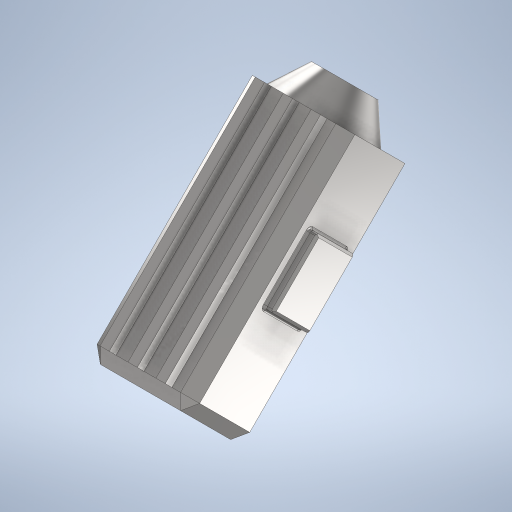
# Autodesk Inventor part: screwdriver
Saved by Autodesk Inventor 2023 (Build 270158000, 158)
## iProperties
Created: 2023-11-21
Part Number: screwdriver
Material: Steel, Mild
Document SubType Name: Modeling
Designer: Beatrice
Density: 7.85 g/cm^3
Appearance: Semi-Polished
Author: Beatrice
Autodesk Inventor part; units mm, degrees
ref_plane "YZ Plane" through (0, 0, 0) normal (1, 0, 0) x (0, 1, 0)
ref_plane "XZ Plane" through (0, 0, 0) normal (0, 1, 0) x (-1, 0, 0)
sketch "Sketch1" plane through (0, 0, 0) normal (1, 0, 0) x (0, 1, 0)
  line L0 (-19.1091, 33.3894) -> (19.1091, 33.3894) construction
  line L1 (-2.4562, 42.2517) -> (-3.9425, 12.3724) construction
  line L2 (-15.9499, 49.3393) -> (15.9499, 17.4395) construction
  line L3 (-15.9953, 17.3941) -> (15.9953, 49.3847) construction
  line L4 (-4.2099, 47.2514) -> (-6.25, 6.2414) construction
  line L5 (17.609, 51.9698) -> (-38.9081, 36.826) construction
  line L6 (18.2302, 47.2514) -> (-40.2807, 47.2514) construction
  line L7 (-2.4567, 42.2414) -> (2.4677, 42.2414) construction
  circle A0 centre (0, 47.2514) radius 3 construction
  ellipse E0 centre (0, 47.2514) end of major axis (4.2185, 47.2514) minor radius 4.2127 (4.2185, 47.2514) -> (-4.2185, 47.2514) ccw construction
  circle A1 centre (0, 47.2514) radius 4.2185 construction
  line L8 (2.4672, 42.2517) -> (-2.4562, 42.2517) construction
  line L9 (4.2215, 47.2514) -> (6.2448, 6.4952) construction
  line L10 (2.4672, 42.2517) -> (3.9506, 12.3724) construction
  line L11 (0.0006, 41.0008) -> (0, 41.0008) construction
  line L12 (-1.0918, 51.3262) -> (1.0918, 43.1767) construction
  line L13 (1.0918, 43.1767) -> (-27.4928, 38.1364) construction
  line L14 (0, 43.0329) -> (-28.9151, 45.5627) construction
  line L15 (-1.0918, 51.3262) -> (-28.367, 41.3989) construction
  line L16 (0, 51.4699) -> (-28.9151, 48.9402) construction
  line L17 (0.0006, 41.0001) -> (0, 41.0001) construction
  ellipse E1 centre (0, 47.2514) end of major axis (-3, 47.2514) minor radius 3 (0.0225, 44.2515) -> (-0.0225, 44.2515) ccw construction
  line L18 (-4.2185, 47.2514) -> (-4.2099, 47.2514) construction
  line L19 (-3.9425, 12.3724) -> (3.9506, 12.3724) construction
  ellipse E2 centre (0, 6.2414) end of major axis (6.25, 6.2414) minor radius 6.2414 (-6.2423, 6.5518) -> (6.2393, 6.6057) ccw construction
  ellipse E3 centre (0, 6.2414) end of major axis (-5, 6.2414) minor radius 5 construction
  line L20 (-6.0016, 11.2344) -> (6.0096, 11.2344) construction
  line L21 (3, 47.2514) -> (4.2185, 47.2514) construction
  line L22 (0, 48.3894) -> (0, 48.3894) construction
  line L23 (0, 51.4699) -> (0, 43.0329) construction
  line L24 (-28.9151, 45.5627) -> (-28.9151, 48.9402) construction
  line L25 (-9.1941, 44.3513) -> (-8.3969, 45.6327) construction
  circle A2 centre (-9.1612, 46.1081) radius 0.5 construction
  circle A3 centre (-9.1612, 46.1081) radius 0.9 construction
  line L26 (-9.1941, 44.3513) -> (-10.078, 43.4674) construction
  line L27 (-10.9619, 46.119) -> (-9.6062, 46.8904) construction
  line L28 (-10.9619, 46.119) -> (-9.1941, 44.3513) construction
  line L29 (-10.9619, 42.5835) -> (-10.078, 43.4674) construction
  line L30 (-11.8457, 45.2351) -> (-10.9619, 46.119) construction
  line L31 (-11.8457, 45.2351) -> (-12.7296, 44.3513) construction
  line L32 (-12.7296, 44.3513) -> (-10.9619, 42.5835) construction
  line L33 (-10.9619, 42.5835) -> (-12.2433, 41.7864) construction
  line L34 (-12.7296, 44.3513) -> (-13.501, 42.9956) construction
  line L35 (-13.4028, 41.8664) -> (-9.1612, 46.1081) construction
  circle A4 centre (-12.7187, 42.5506) radius 0.5 construction
  circle A5 centre (-12.7187, 42.5506) radius 0.9 construction
  line L36 (-27.4928, 38.1364) -> (-28.367, 41.3989) construction
  line L37 (-21.5614, 39.1823) -> (-22.7073, 43.4588) construction
  line L38 (-27.6711, 38.8017) -> (-21.8755, 40.3546) construction
  line L39 (-28.1887, 40.7336) -> (-22.3931, 42.2865) construction
  line L40 (-34.0028, 47.2514) -> (-25.2783, 38.5269) construction
  line L41 (-28.1887, 40.7336) -> (-33.0183, 39.4395) construction
  line L42 (-33.0183, 39.4395) -> (-32.5007, 37.5076) construction
  line L43 (-32.5007, 37.5076) -> (-27.6711, 38.8017) construction
  circle A6 centre (-32.7595, 38.4736) radius 1.01 construction
  circle A7 centre (-32.7595, 38.4736) radius 0.6398 construction
  line L44 (-42.8892, 48.6033) -> (-22.6298, 28.3438) construction
  circle A8 centre (-32.7595, 38.4736) radius 0.6398
  circle A9 centre (-32.7595, 38.4736) radius 1.25
  line L45 (-33.6434, 39.3574) -> (-31.8756, 37.5897)
  line L46 (-31.8756, 37.5897) -> (-33.2898, 36.1755)
  line L47 (-33.2898, 36.1755) -> (-35.0576, 37.9432)
  line L48 (-35.0576, 37.9432) -> (-33.6434, 39.3574)
  circle A10 centre (-33.0183, 39.4395) radius 0.2
  circle A11 centre (-33.7254, 38.2147) radius 0.2
  circle A12 centre (-32.5007, 37.5076) radius 0.2
  circle A13 centre (-31.7936, 38.7324) radius 0.2
  line L49 (-31, 33.8856) -> (-41.6066, 44.4922)
  line L50 (-44.7369, 41.362) -> (-34.1303, 30.7554)
  line L51 (-34.1303, 30.7554) -> (-31, 33.8856)
  line L52 (-33.6434, 39.3574) -> (-35.4365, 38.3222)
  line L53 (-33.6434, 39.3574) -> (-31.5728, 39.3574) construction
  line L54 (-31.8756, 37.5897) -> (-32.9109, 35.7965)
  line L55 (-35.4365, 38.3222) -> (-32.9109, 35.7965)
  line L56 (-32.9109, 35.7965) -> (-33.8666, 34.8408)
  line L57 (-33.8666, 34.8408) -> (-36.3923, 37.3664)
  line L58 (-36.3923, 37.3664) -> (-35.4365, 38.3222)
  line L59 (-41.6066, 44.4922) -> (-44.7369, 41.362)
  line L60 (-43.1717, 42.9271) -> (-32.5651, 32.3205) construction
  line L61 (-43.1717, 42.9271) -> (-45.2366, 44.992) construction
  line L62 (-33.5967, 46.8453) -> (-44.9671, 35.4748) construction
  circle A14 centre (-40.3433, 40.0987) radius 0.85
  line L63 (-50.4924, 41.0001) -> (-32.6081, 23.1158) construction
  line L64 (-50.4924, 41.0001) -> (-25.2002, 41.0001) construction
  line L65 (-46.7349, 37.2426) -> (-43.1994, 33.7071)
  line L66 (-43.1994, 33.7071) -> (-34.4479, 42.4585)
  line L67 (-34.4479, 42.4585) -> (-37.9835, 45.994)
  line L68 (-37.9835, 45.994) -> (-46.7349, 37.2426)
  line L69 (-37.9835, 45.994) -> (-36.14, 46.3809)
  line L70 (-36.14, 46.3809) -> (-35.1005, 45.3414)
  line L71 (-35.1005, 45.3414) -> (-36.6557, 43.7863)
  point P0 (0, 0)
  point P1 (0, 0)
  point P2 (0, 33.3894)
  point P3 (0, 12.3724)
  point P4 (-6.009, 41)
  point P5 (0, 47.2514)
  point P6 (0, 0)
  point P7 (0, 47.2514)
  point P8 (28.7519, 36.3712)
  point P9 (-36.2157, 44.2263)
  dimension "d12" = 3
  dimension "d13" = 5
  dimension "d14" = 6.2414
  dimension "d4" = 41.01
  dimension "d5" = 6.2414
  dimension "d6" = 4.993
  dimension "d7" = 5.69
  dimension "d8" = 29.869
  dimension "d9" = 1.138
  dimension "d10" = 2
  dimension "d11" = 90
  dimension "d15" = 15
  dimension "d16" = 2.5
  dimension "d17" = 1.25
  dimension "d18" = 60
  dimension "d19" = 2
  dimension "d20" = 1
  dimension "d21" = 6
  dimension "d22" = 1
  dimension "d23" = 1.8
  dimension "d24" = 5
  dimension "d25" = 2
  dimension "d26" = 2.02
  dimension "d27" = 2.5
  dimension "d28" = 0.4
  dimension "d29" = 360
  dimension "d30" = 150
  dimension "d31" = 15
  dimension "d32" = 15
  dimension "d33" = 4
  dimension "d34" = 1.7
  dimension "d35" = 45
  dimension "d41" = 2.5
  dimension "d42" = 2.5
  constraints: 144 end point, 30 point on line, 17 parallel, 14 centre point, 12 coincident, 11 perpendicular, 8 midpoint, 7 symmetric about line, 6 point on circle, 4 horizontal, 3 collinear, 2 equal length, 2 horizontal alignment, 2 tangent, 1 concentric, 1 vertical alignment, 49 other
  measures "d4" distance of point (0, 47.251) point (0, 6.241)
  measures "d5" distance of point (0, 0) point (0, 6.241)
  measures "d6" distance from line of point (0, 6.241) L20
  measures "d7" angle of L4 L9
  measures "d8" distance between parallel lines of L19 L7
  measures "d9" distance between parallel lines of L20 L19
  measures "d10" distance between parallel lines of L4 L1
  measures "d11" angle of L2 L3
  measures "d16" distance between parallel lines of L31 L29
  measures "d17" distance between parallel lines of L2 L32
  measures "d18" angle of L40 L5
  measures "d19" distance between parallel lines of L38 L39
  measures "d20" distance between parallel lines of L39 L5
  measures "d21" distance between parallel lines of L37 L36
  measures "d22" diameter of A2
  measures "d23" diameter of A3
  measures "d24" distance between parallel lines of L42 L36
  measures "d25" distance of L46.start L47.start
  measures "d26" diameter of A6
  measures "d27" diameter of A9
  measures "d28" diameter of A10
  measures "d30" angle of L52 L53
  measures "d31" angle of L54 L46
  measures "d32" distance between parallel lines of L51 L59
  measures "d33" distance between parallel lines of L62 L59
  measures "d34" diameter of A14
  measures "d35" angle of L63 L64
  measures "d41" distance between parallel lines of L62 L68
  measures "d42" distance between parallel lines of L66 L62
extrude "Extrusion1" add sketch "Sketch1" against normal blind 2.5 contours L66 L50 L68 L49 | L49 L68 L67 L66 | L66 L65 L68 L50
extrude "Extrusion2" add sketch "Sketch1" along normal blind 3 contours L66 L50 L68 L49 | L49 L68 L67 L66 | L66 L65 L68 L50 | A14
revolve "Revolution1" add sketch "Sketch1" angle 360 about axis through (0, -33.5967, 46.8453) along (0, -0.7071068, -0.7071068) contours L69 L70 L71 L67
chamfer "Chamfer1" distance 0.6 angle 45 8 edges at (3, -38.8236, 38.0828) (-2.5, -38.8236, 38.0828) (3, -42.3592, 41.6183) (-2.5, -42.3592, 41.6183) (0.25, -46.7349, 37.2426) (3, -44.9671, 35.4748) (0.25, -43.1994, 33.7071) (-2.5, -44.9671, 35.4748)
sketch "Sketch2" plane through (0, -35.1005, 45.3414) normal (0, 0.7071068, 0.7071068) x (1, 0, 0)
  circle A0 centre (0, 0) radius 1
  line L0 (0, 1.6487) -> (0, -2)
  line L1 (0, 1.1835) -> (-0.2, 1.1835)
  line L2 (-0.2, 1.1835) -> (-0.2, 0.9798)
  line L3 (0, 1.1835) -> (0.2, 1.1835)
  line L4 (0.2, 1.1835) -> (0.2, 0.9798)
  line L5 (-1.1249, 0.4185) -> (-0.9485, 0.3167)
  line L6 (-1.0249, 0.5917) -> (-1.1249, 0.4185)
  line L7 (-1.0249, 0.5917) -> (-0.9249, 0.765)
  line L8 (-0.9249, 0.765) -> (-0.7485, 0.6631)
  line L9 (-0.9249, -0.765) -> (-0.7485, -0.6631)
  line L10 (-1.0249, -0.5917) -> (-0.9249, -0.765)
  line L11 (-1.0249, -0.5917) -> (-1.1249, -0.4185)
  line L12 (-1.1249, -0.4185) -> (-0.9485, -0.3167)
  line L13 (0.2, -1.1835) -> (0.2, -0.9798)
  line L14 (0, -1.1835) -> (0.2, -1.1835)
  line L15 (0, -1.1835) -> (-0.2, -1.1835)
  line L16 (-0.2, -1.1835) -> (-0.2, -0.9798)
  line L17 (1.1249, -0.4185) -> (0.9485, -0.3167)
  line L18 (1.0249, -0.5917) -> (1.1249, -0.4185)
  line L19 (1.0249, -0.5917) -> (0.9249, -0.765)
  line L20 (0.9249, -0.765) -> (0.7485, -0.6631)
  line L21 (0.9249, 0.765) -> (0.7485, 0.6631)
  line L22 (1.0249, 0.5917) -> (0.9249, 0.765)
  line L23 (1.0249, 0.5917) -> (1.1249, 0.4185)
  line L24 (1.1249, 0.4185) -> (0.9485, 0.3167)
  point P0 (0, 56.8811)
  point P1 (-0.7485, 0.6631)
  point P2 (-0.9485, 0.3167)
  point P3 (-0.9485, -0.3167)
  point P4 (-0.7485, -0.6631)
  point P5 (-0.2, -0.9798)
  point P6 (0.2, -0.9798)
  point P7 (0.7485, -0.6631)
  point P8 (0.9485, -0.3167)
  point P9 (0.9485, 0.3167)
  point P10 (0.7485, 0.6631)
  point P11 (0.2, 0.9798)
  dimension "d46" = 0.2
  dimension "d49" = 360
  constraints: 50 end point, 2 symmetric about line, 1 horizontal, 1 perpendicular, 1 point on line, 58 other
  measures "d46" distance of L1.start L1.end
extrude "Extrusion3" cut sketch "Sketch2" against normal blind 3
sketch "Sketch3" plane through (0, -37.2218, 43.2201) normal (0, 0.7071068, 0.7071068) x (1, 0, 0)
  line L0 (0, 0.85) -> (0, -0.85) projected
  circle A0 centre (0, 0) radius 0.375
  point P0 (0, 56.8811)
  dimension "d53" = 0.75
  constraints: 1 centre point, 1 midpoint
  measures "d53" diameter of A0
extrude "Extrusion4" cut sketch "Sketch3" against normal blind 2
thread "Thread1" size "M0.8x0.2" class "6H" standard "ANSI Metric M Profile" full length
chamfer "Chamfer2" distance 0.125 angle 45 12 edges at (-0.9485, -36.3858, 44.504) (-0.9485, -35.938, 44.0561) (-0.7485, -35.693, 43.8112) (-0.2, -35.4691, 43.5873) (-0.7485, -36.6308, 44.749) (-0.2, -36.8547, 44.9729) (0.2, -35.4691, 43.5873) (0.7485, -35.693, 43.8112) (0.2, -36.8547, 44.9729) (0.7485, -36.6308, 44.749) (0.9485, -35.938, 44.0561) (0.9485, -36.3858, 44.504)
sketch "Sketch4" plane through (0, -35.1005, 45.3414) normal (0, 0.7071068, 0.7071068) x (1, 0, 0)
  line L0 (1.0568, -0.3792) -> (0.9806, -0.1959) projected
  line L1 (1.0568, -0.3792) -> (1.1249, -0.4185) projected
  line L2 (1.1249, -0.4185) -> (0.9249, -0.765) projected
  line L3 (0.9249, -0.765) -> (0.8568, -0.7256) projected
  line L4 (0.66, -0.7513) -> (0.8568, -0.7256) projected
  arc A0 (0.3207, -0.9472) -> (0.66, -0.7513) centre (0, 0) ccw projected
  line L5 (0.2, -1.1048) -> (0.3207, -0.9472) projected
  line L6 (0.2, -1.1048) -> (0.2, -1.1835) projected
  line L7 (0.2, -1.1835) -> (-0.2, -1.1835) projected
  line L8 (-0.2, -1.1835) -> (-0.2, -1.1048) projected
  line L9 (-0.3207, -0.9472) -> (-0.2, -1.1048) projected
  arc A1 (-0.66, -0.7513) -> (-0.3207, -0.9472) centre (0, 0) ccw projected
  line L10 (-0.8568, -0.7256) -> (-0.66, -0.7513) projected
  line L11 (-0.8568, -0.7256) -> (-0.9249, -0.765) projected
  line L12 (-0.9249, -0.765) -> (-1.1249, -0.4185) projected
  line L13 (-1.1249, -0.4185) -> (-1.0568, -0.3792) projected
  line L14 (-0.9806, -0.1959) -> (-1.0568, -0.3792) projected
  arc A2 (-0.9806, 0.1959) -> (-0.9806, -0.1959) centre (0, 0) ccw projected
  line L15 (-1.0568, 0.3792) -> (-0.9806, 0.1959) projected
  line L16 (-1.0568, 0.3792) -> (-1.1249, 0.4185) projected
  line L17 (-1.1249, 0.4185) -> (-0.9249, 0.765) projected
  line L18 (-0.9249, 0.765) -> (-0.8568, 0.7256) projected
  line L19 (-0.66, 0.7513) -> (-0.8568, 0.7256) projected
  arc A3 (-0.3207, 0.9472) -> (-0.66, 0.7513) centre (0, 0) ccw projected
  line L20 (-0.2, 1.1048) -> (-0.3207, 0.9472) projected
  line L21 (-0.2, 1.1048) -> (-0.2, 1.1835) projected
  line L22 (-0.2, 1.1835) -> (0.2, 1.1835) projected
  line L23 (0.2, 1.1835) -> (0.2, 1.1048) projected
  line L24 (0.3207, 0.9472) -> (0.2, 1.1048) projected
  arc A4 (0.66, 0.7513) -> (0.3207, 0.9472) centre (0, 0) ccw projected
  line L25 (0.8568, 0.7256) -> (0.66, 0.7513) projected
  line L26 (0.8568, 0.7256) -> (0.9249, 0.765) projected
  line L27 (0.9249, 0.765) -> (1.1249, 0.4185) projected
  line L28 (1.1249, 0.4185) -> (1.0568, 0.3792) projected
  line L29 (0.9806, 0.1959) -> (1.0568, 0.3792) projected
  arc A5 (0.9806, -0.1959) -> (0.9806, 0.1959) centre (0, 0) ccw projected
  circle A6 centre (0, 0) radius 1.47 projected
  point P0 (0, 56.8811)
thread "Thread2" size "M1.7x0.35" class "6H" standard "ANSI Metric M Profile" full length
sketch "Sketch6" plane through (-1.9, -46.3106, 37.6669) normal (0, -0.7071068, 0.7071068) x (1, 0, 0)
  line L0 (4.3, 11.7764) -> (4.3, 0) projected
  line L1 (1.9, 11.7764) -> (4.3, 11.7764) projected
  line L2 (0, 11.7764) -> (1.9, 11.7764) projected
  line L3 (0, 0) -> (0, 11.7764) projected
  line L4 (4.3, 0) -> (0, 0) projected
  line L5 (0.3362, 11.7764) -> (0.8362, 11.7764)
  line L6 (0.8362, 11.7764) -> (0.8362, 0)
  line L7 (0.8362, 0) -> (0.3362, 0)
  line L8 (0.3362, 0) -> (0.3362, 11.7764)
  line L9 (1.8362, 11.7764) -> (2.3362, 11.7764)
  line L10 (1.8362, 0) -> (1.8362, 11.7764)
  line L11 (2.3362, 11.7764) -> (2.3362, 0)
  line L12 (2.3362, 0) -> (1.8362, 0)
  line L13 (3.3362, 11.7764) -> (3.8362, 11.7764)
  line L14 (3.3362, 0) -> (3.3362, 11.7764)
  line L15 (3.8362, 11.7764) -> (3.8362, 0)
  line L16 (3.8362, 0) -> (3.3362, 0)
  point P0 (1.9, 6.1121)
  dimension "d63" = 0.5
  dimension "d66" = 1.5
  constraints: 24 end point, 2 horizontal, 2 parallel, 2 point on line, 1 perpendicular, 16 other
  measures "d63" distance of L6.end L7.end
  measures "d66" distance of L5.start L9.start
extrude "Extrusion5" add sketch "Sketch6" along normal blind 0.5 contours L15 L4 L14 L1 | L11 L4 L10 L2 L1 | L4 L8 L2 L6
ref_plane "Work Plane1" through (2.4, -44.5429, 35.8991) normal (0, 0.7071068, -0.7071068) x (-1, 0, 0)
mirror "Mirror1" about plane through (2.4, -44.5429, 35.8991) normal (0, 0.7071068, -0.7071068) of "Extrusion5"
sketch "Sketch7" plane through (3, 0, 0) normal (1, 0, 0) x (0, 0, -1)
  line L0 (-42.8828, -34.8722) -> (-34.5556, -43.1994) projected
  line L1 (-42.8828, -34.8722) -> (-45.5698, -37.5592) projected
  line L2 (-37.2426, -45.8864) -> (-45.5698, -37.5592) projected
  line L3 (-34.5556, -43.1994) -> (-37.2426, -45.8864) projected
  line L4 (-45.5698, -37.5592) -> (-37.2426, -45.8864) projected
  line L5 (-43.129, -40) -> (-40.442, -37.313)
  line L6 (-40.442, -37.313) -> (-37.2808, -40.4741)
  line L7 (-37.2808, -40.4741) -> (-39.9678, -43.1611)
  line L8 (-39.9678, -43.1611) -> (-43.129, -40)
  line L9 (-40.442, -38.0201) -> (-42.4219, -40)
  line L10 (-42.4219, -40) -> (-39.9678, -42.454)
  line L11 (-39.9678, -42.454) -> (-37.9879, -40.4741)
  line L12 (-37.9879, -40.4741) -> (-40.442, -38.0201)
  point P0 (0, 0)
  dimension "d74" = 0.5
  constraints: 16 end point, 4 parallel, 3 perpendicular, 2 point on line, 3 other
  measures "d74" distance between parallel lines of L5 L9
extrude "Extrusion6" add sketch "Sketch7" along normal blind 0.5 contours L12 L11 L10 L9
chamfer "Chamfer3" distance 0.125 angle 45 4 edges at (3.5, -39.0101, 41.4319) (3.5, -41.227, 41.1948) (3.5, -41.4641, 38.9779) (3.5, -39.2471, 39.215)
fillet "Fillet1" radius 0.125 8 edges at (3, -41.227, 41.1948) (3, -39.0101, 41.4319) (3, -41.4641, 38.9779) (3, -39.2471, 39.215) (3.1875, -40.4741, 37.9879) (3.1875, -38.0201, 40.442) (3.1875, -42.454, 39.9678) (3.1875, -40, 42.4219)
body "Solid1"
